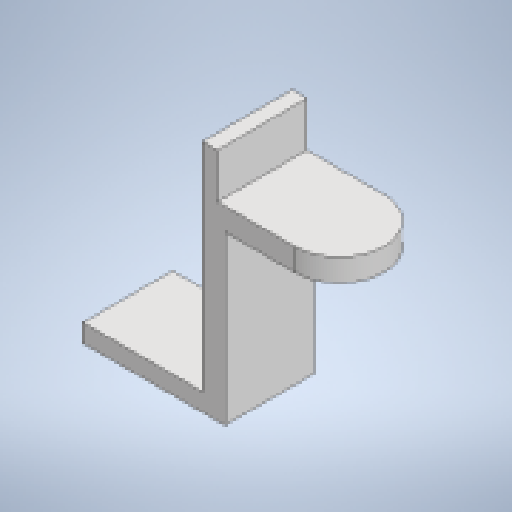
# Autodesk Inventor part: j1 endstop block
Saved by Autodesk Inventor 2025 (Build 290162000, 162)
## iProperties
Created: 2025-07-09
Part Number: j1 endstop block
Material: 一般
Document SubType Name: Modeling
Designer: gavin
Density: 1 g/cm^3
Appearance: 預設
Author: gavin
Autodesk Inventor part; units mm, degrees
ref_plane "YZ Plane" through (0, 0, 0) normal (1, 0, 0) x (0, 1, 0)
ref_plane "XZ Plane" through (0, 0, 0) normal (0, 1, 0) x (-1, 0, 0)
ref_plane "XY Plane" through (0, 0, 0) normal (0, 0, 1) x (1, 0, 0)
sketch "草圖1" plane through (0, 0, 0) normal (0, 0, 1) x (1, 0, 0)
  line L0 (-1.8649, 0) -> (-1.8649, -6) construction
  line L1 (-1.8649, -6) -> (-0.9249, -6) construction
  line L2 (-1.8649, 0) -> (-1.8649, -6) construction
  line L3 (-0.9249, 0) -> (0, 0) projected
  line L4 (-0.9249, 0) -> (-0.9249, -6) construction
  line L5 (2.6286, 0) -> (2.6286, -6)
  line L6 (2.6286, -6) -> (7.6286, -6) projected
  line L7 (7.6286, 0) -> (7.6286, -6)
  line L8 (-1.8949, -3) -> (-0.8949, -3)
  line L9 (-0.8949, -3) -> (-0.8949, -6)
  line L10 (-0.8949, -6) -> (9.1286, -6)
  line L11 (9.1286, -6) -> (9.1286, -7.5)
  line L12 (9.1286, -7.5) -> (-0.3949, -7.5)
  line L13 (-0.3949, -7.5) -> (-0.3949, -20.2)
  line L14 (-0.3949, -20.2) -> (-9.8949, -20.2)
  line L15 (-9.8949, -20.2) -> (-9.8949, -19)
  line L16 (-9.8949, -19) -> (-1.8949, -19)
  line L17 (-1.8949, -19) -> (-1.8949, -3)
  dimension "d0" = 1
  dimension "d1" = 0.03
  dimension "d2" = 1.5
  dimension "d3" = 16
  dimension "d4" = 1.5
  dimension "d5" = 1.5
  dimension "d6" = 8
  dimension "d7" = 1.2
  dimension "d11" = 3
  constraints: 24 end point, 6 vertical, 3 perpendicular, 2 parallel, 1 horizontal, 1 point on line, 3 other
  measures "d0" distance of L8.start L8.end
  measures "d1" distance between parallel lines of L17 L0
  measures "d2" distance between parallel lines of L7 L11
  measures "d3" distance of L16.end L8.start
  measures "d4" distance of L10.end L11.end
  measures "d5" distance between parallel lines of L13 L17
  measures "d6" distance of L15.end L16.end
  measures "d7" distance of L14.end L15.end
  measures "d11" distance of L8.end L9.end
extrude "擠出1" add sketch "草圖1" along normal blind 6
fillet "圓角1" radius 3 2 edges at (9.1286, -6.75, 6) (9.1286, -6.75, 0)
sketch "草圖2" plane through (-0.8949, -6, 6) normal (0, 1, 0) x (1, 0, 0)
  circle A0 centre (4.97, 3) radius 1.5 projected
  point P0 (0.8949, 6)
extrude "擠出2" cut sketch "草圖2" against normal up to surface (1.5 mm away)
fillet "圓角2" radius 1.5 2 edges at (-1.8949, -19, 3) (-0.3949, -20.2, 3)
